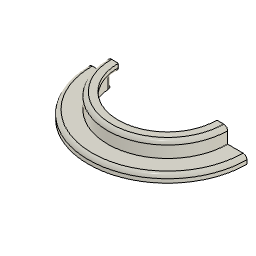
UrinSensorHalter (Autodesk Fusion 360 design; units mm, degrees)
Autodesk Fusion 360 part; units mm, degrees
sketch "Skizze2" plane through (0, 0, 0) normal (0, 0, 1) x (1, 0, 0)
  circle A0 centre (0, 0) radius 15.5
  circle A1 centre (0, 0) radius 12.75
  circle A2 centre (0, 0) radius 20.5
  circle A3 centre (0, 0) radius 14.25
  dimension "d4" = 31
  dimension "d5" = 25.5
  dimension "d6" = 41
  dimension "d37" = 28.5
  constraint coincident A0.centre A1.centre
  constraint concentric A0 A3
  measures "d4" diameter of A0
  measures "d5" diameter of A1
  measures "d6" diameter of A2
  measures "d37" diameter of A3
extrude "Extrusion15" add sketch "Skizze2" along normal blind 2 contours A2 makes body 1
sketch "Skizze7" plane through (0, 0, 0) normal (0, 0, 1) x (1, 0, 0)
  line L0 (-24, 0) -> (26, 0)
  line L1 (26, 0) -> (26, 23)
  line L2 (26, 23) -> (-24, 23)
  line L3 (-24, 23) -> (-24, 0)
  constraint horizontal L0
  constraint vertical L1
  constraint horizontal L2
  constraint vertical L3
extrude "Extrusion12" add sketch "Skizze2" along normal blind 2 separate body contours A2 makes body 2
extrude "Extrusion13" add sketch "Skizze2" along normal blind 6 contours A0 | A3 bodies 2
extrude "Extrusion16" cut sketch "Skizze2" along normal blind 4 contours A3 bodies 2
extrude "Extrusion17" cut sketch "Skizze7" along normal blind 10 bodies 1 2
fillet "Abrundung1" radius 1 1 edges at (0, -15.5, 6) on bodies 2
fillet "Abrundung2" radius 1 1 edges at (0, -20.5, 2) on bodies 2
fillet "Abrundung3" radius 1 1 edges at (0, -20.5, 2) on bodies 1
fillet "Abrundung4" radius 1 1 edges at (0, -12.75, 4) on bodies 2
fillet "Abrundung5" radius 1.3 1 edges at (14.25, 0, 2) on bodies 2
fillet "Abrundung6" radius 1.3 1 edges at (-14.25, 0, 2) on bodies 2
extrude "Extrusion9" [rolled back] along distance 16 taper angle 0
extrude "Extrusion10" [rolled back] along distance 11 taper angle 0
